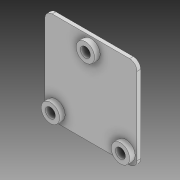
# Autodesk Inventor part: J0_EncoderBracket
Saved by Autodesk Inventor 2020 (Build 240168000, 168)
## iProperties
Created: 2021-06-12
Part Number: J0_EncoderBracket
Material: Generic
Document SubType Name: Modeling
Designer: DDeGo
Density: 1 g/cm^3
Appearance: Default
Author: DDeGo
Autodesk Inventor part; units mm, degrees
ref_plane "YZ Plane" through (0, 0, 0) normal (1, 0, 0) x (0, 1, 0)
ref_plane "XZ Plane" through (0, 0, 0) normal (0, 1, 0) x (-1, 0, 0)
ref_plane "XY Plane" through (0, 0, 0) normal (0, 0, 1) x (1, 0, 0)
sketch "Sketch1" plane through (0, 0, 0) normal (0, 0, 1) x (1, 0, 0)
  line L0 (-10.5, -12.5) -> (10.5, -12.5)
  line L1 (12.5, -10.5) -> (12.5, 10.5)
  line L2 (10.5, 12.5) -> (-10.5, 12.5)
  line L3 (-12.5, 10.5) -> (-12.5, -10.5)
  line L4 (-12.5, -12.5) -> (12.5, 12.5) construction
  line L5 (12.5, -12.5) -> (-12.5, 12.5) construction
  line L6 (0, 0) -> (0, 9.5) construction
  line L7 (0, 0) -> (0, -9.5) construction
  line L8 (0, -9.5) -> (-9.5, -9.5) construction
  line L9 (0, -9.5) -> (9.5, -9.5) construction
  circle A0 centre (-9.5, -9.5) radius 1.35
  circle A1 centre (9.5, -9.5) radius 1.35
  circle A2 centre (0, 9.5) radius 1.35
  arc A3 (-10.5, 12.5) -> (-12.5, 10.5) centre (-10.5, 10.5) ccw
  arc A4 (12.5, 10.5) -> (10.5, 12.5) centre (10.5, 10.5) ccw
  arc A5 (10.5, -12.5) -> (12.5, -10.5) centre (10.5, -10.5) ccw
  arc A6 (-12.5, -10.5) -> (-10.5, -12.5) centre (-10.5, -10.5) ccw
  dimension "d0" = 25
  dimension "d1" = 25
  dimension "d2" = 19
  dimension "d3" = 19
  dimension "d4" = 2.7
  dimension "d7" = 2
  constraints: 20 end point, 8 point on circle, 8 point on line, 8 tangent, 7 centre point, 5 equal radius, 3 coincident, 2 collinear, 2 horizontal, 2 midpoint, 2 parallel, 2 perpendicular, 2 vertical
  measures "d0" distance of L4.start L5.start
  measures "d1" distance of L5.start L4.end
  measures "d2" distance of L6.end L7.end
  measures "d3" distance of L9.end L8.end
  measures "d4" diameter of A0
  measures "d7" radius of A3
extrude "Extrusion1" add sketch "Sketch1" along normal blind 1
sketch "Sketch2" plane through (0, 0, 1) normal (0, 0, 1) x (1, 0, 0)
  circle A0 centre (0, 9.5) radius 1.35 projected
  circle A1 centre (0, 9.5) radius 2.5
  circle A2 centre (9.5, -9.5) radius 1.35 projected
  circle A3 centre (9.5, -9.5) radius 2.5
  circle A4 centre (-9.5, -9.5) radius 1.35 projected
  circle A5 centre (-9.5, -9.5) radius 2.5
  point P0 (0, 0)
  dimension "d8" = 5
  constraints: 3 centre point, 3 coincident, 2 equal radius
  measures "d8" diameter of A1
extrude "Extrusion2" add sketch "Sketch2" along normal blind 1.5
body "Solid1"
